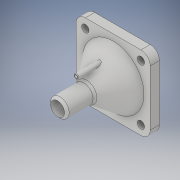
# Autodesk Inventor part: FrameToPipe
Saved by Autodesk Inventor 2018 (Build 220112000, 112)
## iProperties
Created: 2020-03-23
Part Number: FrameToPipe
Material: Generic
Document SubType Name: Modeling
Designer: emile
Density: 1 g/cm^3
Appearance: Default
Author: emile
Autodesk Inventor part; units mm, degrees
ref_plane "YZ Plane" through (0, 0, 0) normal (1, 0, 0) x (0, 1, 0)
ref_plane "XZ Plane" through (0, 0, 0) normal (0, 1, 0) x (-1, 0, 0)
sketch "Sketch26" plane through (0, 0, 0) normal (0, 0, 1) x (1, 0, 0)
  line L0 (-50.8, 0) -> (-50.8, -50.8)
  line L1 (-50.8, -50.8) -> (50.8, -50.8)
  line L2 (50.8, -50.8) -> (50.8, 0)
  circle A0 centre (0, 0) radius 42.2275
  arc A1 (50.8, 0) -> (-50.8, 0) centre (0, 0) ccw
  arc A2 (-0.1798, -50.8) -> (0.1798, -50.8) centre (0, 0) ccw
  line L3 (-50.8, 0) -> (-50.8, 50.8)
  line L4 (-50.8, 50.8) -> (0, 50.8)
  dimension "d127" = 50.8
  dimension "d128" = 101.6
  dimension "d129" = 84.455
  constraints: 10 end point, 6 point on circle, 3 centre point, 3 perpendicular, 3 point on line, 3 tangent, 2 coincident, 2 vertical, 1 parallel
  measures "d127" distance from line of L1 point (0, 0)
  measures "d128" distance of L0.end L1.end
  measures "d129" diameter of A0
ref_plane "Work Plane3" through (0, 0, 38.1) normal (0, 0, 1) x (1, 0, 0)
sketch "Sketch27" plane through (0, 0, 38.1) normal (0, 0, 1) x (1, 0, 0)
  circle A0 centre (0, 0) radius 12.7
  dimension "d131" = 25.4
  constraints: 1 centre point, 1 coincident
  measures "d131" diameter of A0
loft "Loft2" add profiles "Sketch27", "Sketch26" contours all / A0
shell "Shell2" thickness 3.81 removed faces 2 at (-16.9418, 16.4631, 0) at (-3.6254, -0.9542, 38.1)
sketch "Sketch28" plane through (0, 0, 0) normal (0, 0, -1) x (-1, 0, 0)
  line L0 (-50.8, -50.8) -> (-50.8, 0) projected
  arc A0 (50.8, 0) -> (-50.8, 0) centre (0, 0) ccw projected
  circle A1 centre (0, 0) radius 42.2275 projected
  circle A2 centre (0, 0) radius 37.4072 projected
  circle A3 centre (0, 0) radius 37.4072 projected
  circle A4 centre (0, 0) radius 42.2275 projected
  line L1 (50.8, -50.8) -> (-50.8, -50.8) projected
  line L2 (50.8, 0) -> (50.8, -50.8) projected
extrude "Extrusion31" add sketch "Sketch28" along normal blind 12.7 contours L0 A0 L2 L1 | A1
fillet "Fillet5" radius 25.4 2 edges at (0, 37.4072, 0) (0, -37.4072, 0)
sketch "Sketch29" plane through (0, 0, 38.1) normal (0, 0, 1) x (1, 0, 0)
  circle A0 centre (0, 0) radius 7.8797 projected
  circle A1 centre (0, 0) radius 12.7 projected
  circle A2 centre (0, 0) radius 9.525
  dimension "d144" = 19.05
  constraints: 1 centre point, 1 coincident
  measures "d144" diameter of A2
extrude "Extrusion32" cut sketch "Sketch29" against normal through all contours A2
sketch "Sketch31" plane through (0, 0, -12.7) normal (0, 0, -1) x (-1, 0, 0)
  circle A0 centre (0, 0) radius 12.7
  circle A1 centre (0, 0) radius 7.9375
  circle A2 centre (0, 0) radius 6.4135
  line L0 (12.2967, 3.175) -> (12.2967, -3.175)
  line L1 (12.2967, -3.175) -> (37.4072, -3.175)
  line L2 (37.4072, -3.175) -> (37.4072, 3.175)
  line L3 (37.4072, 3.175) -> (12.2967, 3.175)
  circle A3 centre (0, 0) radius 37.4072 projected
  point P0 (37.4072, 0)
  point P1 (12.2967, 0)
  dimension "d147" = 25.4
  dimension "d148" = 15.875
  dimension "d149" = 12.827
  dimension "d150" = 6.35
  constraints: 8 end point, 3 coincident, 2 centre point, 2 horizontal alignment, 2 midpoint, 2 parallel, 1 perpendicular, 1 vertical, 4 other
  measures "d148" diameter of A1
  measures "d149" diameter of A2
  measures "d150" distance of L0.start L0.end
extrude "Extrusion33" add sketch "Sketch31" against normal blind 12.7 contours A0 L0 | A0 L3 A3 L1 | L3 L2 A3 | A3 L2 L1 picked at (12.3712, -0.7098) picked at (20.9157, 0.7093)
extrude "Extrusion34" add sketch "Sketch31" against normal blind 12.7 contours A0 L0 | L0 A0 | A1
extrude "Extrusion35" cut sketch "Sketch31" against normal blind 5.08 contours A1
fillet "Fillet6" radius 6.35 6 edges at (-12.2967, 3.175, -6.35) (-12.2967, -3.175, -6.35) (-37.2723, 3.175, -10.6952) (-36.8898, 3.175, -4.3072) (-36.8898, -3.175, -4.3072) (-37.2723, -3.175, -10.6952)
pattern_circular "Circular Pattern4" count 2 over 360 about axis through (0, 0, -12.7) along (0, 0, 1) of "Extrusion33", "Fillet6"
sketch "Sketch32" plane through (0, 0, 38.1) normal (0, 0, 1) x (1, 0, 0)
  circle A0 centre (0, 0) radius 9.525 projected
  circle A1 centre (0, 0) radius 12.7 projected
extrude "Extrusion36" add sketch "Sketch32" along normal blind 38.1
fillet "Fillet7" radius 6.35 1 edges at (-12.7, 0, 38.1)
chamfer "Chamfer5" distance 3.175 angle 45 1 edges at (-12.7, 0, 76.2)
sketch "Sketch33" plane through (0, 0, 38.1) normal (0, 0, 1) x (1, 0, 0)
  circle A0 centre (0, 25.4) radius 3.175
  circle A1 centre (0, 0) radius 32.0838 projected
  circle A2 centre (0, 25.4) radius 1.905
  dimension "d167" = 25.4
  dimension "d168" = 6.35
  dimension "d169" = 1.27
  constraints: 2 centre point, 1 coincident, 1 vertical alignment
  measures "d167" distance of A1.centre A0.centre
  measures "d168" diameter of A0
  measures "d169" radial gap between concentric circles of A0 A2
extrude "Extrusion37" add sketch "Sketch33" against normal up to surface contours A0 round surface about axis through (0, 0, 0) along (0, 0, 1) radius 42.2275 half angle -37.775684 far side no
extrude "Extrusion38" cut sketch "Sketch33" against normal through all contours A2
extrude "Extrusion39" add sketch "Sketch33" along normal blind 12.7 contours A0
chamfer "Chamfer6" distance 0.635 angle 45 1 edges at (-3.175, 25.4, 50.8)
extrude "Extrusion40" add sketch "Sketch26" against normal up to surface (12.7 mm away) contours L3 L4 A1
sketch "Sketch34" plane through (0, 0, 0) normal (0, 0, 1) x (1, 0, 0)
  point P0 (-38.1, 38.1)
  point P1 (-38.1, -38.1)
  point P2 (38.1, -38.1)
  point P3 (38.1, 38.1)
hole "Hole1" at (-38.1, 38.1, 0) at (-38.1, -38.1, 0) at (38.1, -38.1, 0) at (38.1, 38.1, 0) direction (0, 0, -1) diameter 10.0838 depth 12.7
sketch "Sketch35" plane through (0, 0, 0) normal (0, 0, 1) x (1, 0, 0)
  arc A0 (50.8, 0) -> (0, 50.8) centre (0, 0) ccw projected
  line L0 (50.8, 0) -> (50.8, -25.4)
  line L1 (50.8, -25.4) -> (50.8, 0)
  line L2 (50.8, 0) -> (50.8, -25.4)
  line L3 (50.8, 0) -> (50.8, -50.8) projected
  line L4 (50.8, 0) -> (50.8, -25.4)
  line L5 (50.8, 0) -> (50.8, 50.8)
  line L6 (50.8, 50.8) -> (0, 50.8)
  constraints: 12 end point, 3 tangent, 2 collinear, 1 perpendicular, 1 point on line
extrude "Extrusion41" add sketch "Sketch35" against normal up to surface (12.7 mm away)
sketch "Sketch36" plane through (0, 0, 0) normal (0, 0, 1) x (1, 0, 0)
  circle A0 centre (-38.1, -38.1) radius 5.0419 projected
  circle A1 centre (-38.1, 38.1) radius 5.0419 projected
  circle A2 centre (38.1, -38.1) radius 5.0419 projected
  line L0 (50.8, -50.8) -> (-50.8, -50.8) projected
  line L1 (50.8, -50.8) -> (50.8, 50.8) projected
  line L2 (50.8, 50.8) -> (-50.8, 50.8) projected
  line L3 (-50.8, -50.8) -> (-50.8, 50.8) projected
  circle A3 centre (0, 0) radius 42.2275 projected
  circle A4 centre (38.1, 38.1) radius 5.0419
  circle A5 centre (38.1, -38.1) radius 5.0419 projected
  constraints: 1 centre point, 1 equal radius, 1 horizontal alignment, 1 vertical alignment
extrude "Extrusion42" cut sketch "Sketch36" against normal through all contours A4
fillet "Fillet8" radius 12.7 4 edges at (-50.8, 50.8, -6.35) (50.8, 50.8, -6.35) (50.8, -50.8, -6.35) (-50.8, -50.8, -6.35)
body "Solid2"
